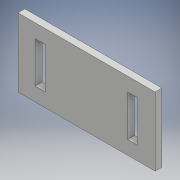
# Autodesk Inventor part: Base
Saved by Autodesk Inventor 2017 SP1 (Build 210196100, 196)
## iProperties
Part Number: Base
Material: Générique
Document SubType Name: Modeling
Designer: Sylvain
Density: 1 g/cm^3
Appearance: Par défaut
Author: Sylvain
Autodesk Inventor part; units mm, degrees
ref_plane "YZ Plane" through (0, 0, 0) normal (1, 0, 0) x (0, 1, 0)
ref_plane "XZ Plane" through (0, 0, 0) normal (0, 1, 0) x (-1, 0, 0)
ref_plane "XY Plane" through (0, 0, 0) normal (0, 0, 1) x (1, 0, 0)
sketch "Esquisse1" plane through (0, 0, 0) normal (0, 1, 0) x (-1, 0, 0)
  line L0 (0, 0) -> (200, 0)
  line L1 (200, 0) -> (200, -100)
  line L2 (200, -100) -> (0, -100)
  line L3 (0, -100) -> (0, 0)
  dimension "d0" = 200
  dimension "d1" = 100
  constraints: 8 end point, 2 parallel, 1 horizontal, 1 perpendicular
  measures "d0" distance of L1.end L2.end
  measures "d1" distance of L0.end L1.end
extrude "Extrusion1" add sketch "Esquisse1" along normal blind 10
sketch "Esquisse2" plane through (0, 10, 0) normal (0, 1, 0) x (1, 0, 0)
  line L0 (-175, 80) -> (-160, 80)
  line L1 (-160, 80) -> (-160, 20)
  line L2 (-160, 20) -> (-175, 20)
  line L3 (-175, 20) -> (-175, 80)
  line L4 (-40, 80) -> (-25, 80)
  line L5 (-25, 80) -> (-25, 20)
  line L6 (-25, 20) -> (-40, 20)
  line L7 (-40, 20) -> (-40, 80)
  line L8 (-200, 0) -> (0, 0) projected
  line L9 (-200, 100) -> (-200, 0) projected
  line L10 (0, 0) -> (0, 100) projected
  dimension "d4" = 60
  dimension "d5" = 15
  dimension "d6" = 60
  dimension "d7" = 15
  dimension "d8" = 20
  dimension "d9" = 25
  dimension "d10" = 25
  constraints: 16 end point, 4 parallel, 2 horizontal, 2 perpendicular, 1 point on line
  measures "d4" distance between parallel lines of L2 L0
  measures "d5" distance between parallel lines of L1 L3
  measures "d6" distance between parallel lines of L6 L4
  measures "d7" distance between parallel lines of L5 L7
  measures "d8" distance between parallel lines of L8 L2
  measures "d9" distance between parallel lines of L9 L3
  measures "d10" distance between parallel lines of L10 L5
extrude "Extrusion2" cut sketch "Esquisse2" against normal blind 10
